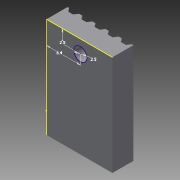
# Autodesk Inventor part: belt clamp
Saved by Autodesk Inventor 2015 SP1 (Build 190203100, 203)
## iProperties
Created: 2015-04-24
Part Number: belt clamp
Material: Generic
Document SubType Name: Modeling
Designer: ubik
Density: 1 g/cm^3
Appearance: Default
Author: ubik
Autodesk Inventor part; units mm, degrees
ref_plane "YZ Plane" through (0, 0, 0) normal (1, 0, 0) x (0, 1, 0)
ref_plane "XZ Plane" through (0, 0, 0) normal (0, 1, 0) x (-1, 0, 0)
ref_plane "XY Plane" through (0, 0, 0) normal (0, 0, 1) x (1, 0, 0)
sketch "Sketch1" plane through (0, 0, 0) normal (0, 0, 1) x (1, 0, 0)
  line L0 (12.5, 15) -> (12.5, 0)
  line L1 (0, 0) -> (12.5, 0)
  line L2 (0, 15) -> (12.5, 15)
  line L3 (0, 15) -> (0, 0)
  constraints: 9 end point, 1 horizontal, 1 perpendicular
extrude "Extrusion2" add sketch "Sketch1" along normal blind 4
sketch "Sketch2" plane through (0, 0, 0) normal (0, -1, 0) x (1, 0, 0)
  line L0 (12.5, 0) -> (0, 0) projected
  line L1 (12.5, 0) -> (12.5, 4) projected
  line L2 (0, 4) -> (12.5, 4) projected
  line L3 (0, 0) -> (0, 4) projected
extrude "Extrusion3" add sketch "Sketch2" along normal blind 4
sketch "Sketch4" plane through (0, -4, 0) normal (0, -1, 0) x (1, 0, 0)
  line L0 (10, 0) -> (10.1908, 0)
  line L1 (10.359, 0.0918) -> (10.691, 0.6082)
  line L2 (11.809, 0.6082) -> (12.141, 0.0918)
  line L3 (10.8592, 0.7) -> (11.6408, 0.7)
  arc A0 (11.809, 0.6082) -> (11.6408, 0.7) centre (11.6408, 0.5) ccw
  arc A1 (10.8592, 0.7) -> (10.691, 0.6082) centre (10.8592, 0.5) ccw
  line L4 (12.3092, 0) -> (12.5, 0)
  arc A2 (10.1908, 0) -> (10.359, 0.0918) centre (10.1908, 0.2) ccw
  arc A3 (12.141, 0.0918) -> (12.3092, 0) centre (12.3092, 0.2) ccw
  line L5 (7.5, 0) -> (7.6908, 0)
  arc A4 (7.6908, 0) -> (7.859, 0.0918) centre (7.6908, 0.2) ccw
  line L6 (7.859, 0.0918) -> (8.191, 0.6082)
  arc A5 (8.3592, 0.7) -> (8.191, 0.6082) centre (8.3592, 0.5) ccw
  line L7 (8.3592, 0.7) -> (9.1408, 0.7)
  arc A6 (9.309, 0.6082) -> (9.1408, 0.7) centre (9.1408, 0.5) ccw
  line L8 (9.309, 0.6082) -> (9.641, 0.0918)
  arc A7 (9.641, 0.0918) -> (9.8092, 0) centre (9.8092, 0.2) ccw
  line L9 (9.8092, 0) -> (10, 0)
  line L10 (5, 0) -> (5.1908, 0)
  arc A8 (5.1908, 0) -> (5.359, 0.0918) centre (5.1908, 0.2) ccw
  line L11 (5.359, 0.0918) -> (5.691, 0.6082)
  arc A9 (5.8592, 0.7) -> (5.691, 0.6082) centre (5.8592, 0.5) ccw
  line L12 (5.8592, 0.7) -> (6.6408, 0.7)
  arc A10 (6.809, 0.6082) -> (6.6408, 0.7) centre (6.6408, 0.5) ccw
  line L13 (6.809, 0.6082) -> (7.141, 0.0918)
  arc A11 (7.141, 0.0918) -> (7.3092, 0) centre (7.3092, 0.2) ccw
  line L14 (7.3092, 0) -> (7.5, 0)
  line L15 (2.5, 0) -> (2.6908, 0)
  arc A12 (2.6908, 0) -> (2.859, 0.0918) centre (2.6908, 0.2) ccw
  line L16 (2.859, 0.0918) -> (3.191, 0.6082)
  arc A13 (3.3592, 0.7) -> (3.191, 0.6082) centre (3.3592, 0.5) ccw
  line L17 (3.3592, 0.7) -> (4.1408, 0.7)
  arc A14 (4.309, 0.6082) -> (4.1408, 0.7) centre (4.1408, 0.5) ccw
  line L18 (4.309, 0.6082) -> (4.641, 0.0918)
  arc A15 (4.641, 0.0918) -> (4.8092, 0) centre (4.8092, 0.2) ccw
  line L19 (4.8092, 0) -> (5, 0)
  line L20 (0, 0) -> (0.1908, 0)
  arc A16 (0.1908, 0) -> (0.359, 0.0918) centre (0.1908, 0.2) ccw
  line L21 (0.359, 0.0918) -> (0.691, 0.6082)
  arc A17 (0.8592, 0.7) -> (0.691, 0.6082) centre (0.8592, 0.5) ccw
  line L22 (0.8592, 0.7) -> (1.6408, 0.7)
  arc A18 (1.809, 0.6082) -> (1.6408, 0.7) centre (1.6408, 0.5) ccw
  line L23 (1.809, 0.6082) -> (2.141, 0.0918)
  arc A19 (2.141, 0.0918) -> (2.3092, 0) centre (2.3092, 0.2) ccw
  line L24 (2.3092, 0) -> (2.5, 0)
  line L25 (7.3092, 0) -> (7.6908, 0)
  line L26 (9.8092, 0) -> (10.1908, 0)
  line L27 (12.3092, 0) -> (12.5, 0)
  line L28 (4.8092, 0) -> (5.1908, 0)
  line L29 (0, 0) -> (0.1908, 0)
  line L30 (2.3092, 0) -> (2.6908, 0)
  line L31 (12.5, 0) -> (12.5, -1)
  line L32 (12.5, -1) -> (0, -1)
  line L33 (0, -1) -> (0, 0)
  point P0 (0, 0)
  point P1 (0, 0)
  point P2 (10.3, 0)
  point P3 (12.2, 0)
  point P4 (7.8, 0)
  point P5 (9.7, 0)
  point P6 (5.3, 0)
  point P7 (7.2, 0)
  point P8 (2.8, 0)
  point P9 (4.7, 0)
  point P10 (0.3, 0)
  point P11 (2.2, 0)
  dimension "d11" = 0.3
  dimension "d12" = 0.2
  dimension "d13" = 0.2
  dimension "d14" = 2.5
  dimension "d16" = 1
  constraints: 68 end point, 40 point on circle, 20 centre point, 20 point on line, 8 tangent, 6 horizontal, 2 equal radius, 2 perpendicular, 1 vertical
  measures "d11" distance of L0.start point (10.3, 0)
  measures "d12" radius of A0
  measures "d13" radius of A2
  measures "d14" distance of L0.start L5.start
  measures "d16" distance of L27.end L31.end
extrude "Extrusion4" cut sketch "Sketch4" against normal through all
sketch "Sketch5" plane through (0, 0, 4) normal (0, 0, 1) x (1, 0, 0)
  arc A0 (7.3092, 11.7007) -> (7.3092, 13.2993) centre (6.375, 12.5) ccw projected
  circle A1 centre (6.375, 12.5) radius 1.25
  dimension "d19" = 2.5
  constraints: 1 centre point, 1 coincident
  measures "d19" diameter of A1
sketch "Sketch6" plane through (0, 0, 4) normal (0, 0, 1) x (1, 0, 0)
  circle A0 centre (6.4, 12.5) radius 1.25
  line L0 (12.5, 15) -> (0, 15) projected
  line L1 (0, 15) -> (0, -4) projected
  point P0 (0, 0)
  dimension "d20" = 2.5
  dimension "d21" = 2.5
  dimension "d22" = 6.4
  constraints: 1 centre point
  measures "d20" diameter of A0
  measures "d21" distance from line of A0.centre L0
  measures "d22" distance from line of A0.centre L1
extrude "Extrusion5" cut sketch "Sketch5" against normal through all
body "Solid2"
